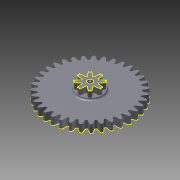
# Autodesk Inventor part: Spur Gear1
Saved by Autodesk Inventor 2014 SP1 (Build 180222100, 222)
## iProperties
Created: 2017-09-24
Part Number: Spur Gear1
Material: Steel
Document SubType Name: Modeling
Designer: Vivi
Categories: <?xml version="1.0" encoding="UTF-16"?> <MemberInstance><Categories><FamilyTemplate><FamilyTemplateParameter ValueType="xs:double" Id="1" ObjectReferenceKey="da_z" ObjectType="kUserParameterObject"/><FamilyTemplateParameter ValueType="xs:double" Id="2" ObjectReferenceKey="da_b" ObjectType="kUserParameterObject"/><FamilyTemplateParameter ValueType="xs:double" Id="3" ObjectReferenceKey="da_beta" ObjectType="kUserParameterObject"/><FamilyTemplateParameter ValueType="xs:double" Id="4" ObjectReferenceKey="da_da" ObjectType="kUserParameterObject"/><FamilyTemplateParameter ValueType="xs:double" Id="5" ObjectReferenceKey="da_aw" ObjectType="kUserParameterObject"/><FamilyTemplateParameter ValueType="xs:string" Id="6" ObjectReferenceKey="EAIAABAAAACIAQAAAAAAAIAAAAAAAAAA" ObjectType="83910656" SubObjectId="SurfaceGeometry"/></FamilyTemplate><ParamToTemplateMap><ParamToTemplate CategoryParameter="//CategoryParameter[@InternalName='046C89C9-8512-4d59-83FE-43B91F4F132A']" TemplateParameter="1"/><ParamToTemplate CategoryParameter="//CategoryParameter[@InternalName='2552DF32-E462-4b46-AEBF-C6C7768E72AC']" TemplateParameter="2"/><ParamToTemplate CategoryParameter="//CategoryParameter[@InternalName='C9EE641D-15FC-4fae-A226-E94C4372FDD7']" TemplateParameter="3"/><ParamToTemplate><ParamToTemplate CategoryParameter="//CategoryParameter[@InternalName='00B6519A-459B-49c7-AD84-2E56D39A5744']" ConstantValue="0.000000"/></ParamToTemplate><ParamToTemplate><ParamToTemplate CategoryParameter="//CategoryParameter[@InternalName='04B31F0E-C7A6-4894-AA32-9629BEFACF47']" ConstantValue="1.000000"/></ParamToTemplate><ParamToTemplate><ParamToTemplate CategoryParameter="//CategoryParameter[@InternalName='43CBEC2E-7847-49e7-A936-2F7889FCB2D9']" ConstantValue="0.250000"/></ParamToTemplate><ParamToTemplate><ParamToTemplate CategoryParameter="//CategoryParameter[@InternalName='B1EFC894-105D-4ebd-86BF-FA20ED196853']" ConstantValue="0.350000"/></ParamToTemplate><ParamToTemplate><ParamToTemplate CategoryParameter="//CategoryParameter[@InternalName='51175063-3D10-4879-93E8-6246FE8B403D']" ConstantValue="2060000000.000000"/></ParamToTemplate><ParamToTemplate><ParamToTemplate CategoryParameter="//CategoryParameter[@InternalName='A3A52E27-4454-46a9-B0BD-C932399B70AF']" ConstantValue="0.300000"/></ParamToTemplate><ParamToTemplate><ParamToTemplate CategoryParameter="//CategoryParameter[@InternalName='91B76062-C214-41d9-B1B9-14D2AB99603D']" ConstantValue="0.150000"/></ParamToTemplate><ParamToTemplate><ParamToTemplate CategoryParameter="//CategoryParameter[@InternalName='374E806E-8B8A-4dda-A9AA-1039D6500AD2']" ConstantValue="6.666667"/></ParamToTemplate><ParamToTemplate><ParamToTemplate CategoryParameter="//CategoryParameter[@InternalName='2D373A89-B862-43d6-8D0B-0CBF12AB9F6C']" ConstantValue="0.523599"/></ParamToTemplate><ParamToTemplate CategoryParameter="//CategoryParameter[@InternalName='37777632-D6A2-4fac-9D53-DB8ACD95C989']" TemplateParameter="4"/><ParamToTemplate CategoryParameter="//CategoryParameter[@InternalName='FD1017F1-B727-4f7e-9707-0F86F1FF9423']" TemplateParameter="5"/><ParamToTemplate><ParamToTemplate CategoryParameter="//CategoryParameter[@InternalName='9E1B4470-B2D3-4ff1-B813-535BB4CDF51A']" ConstantValue="3520000.000000"/></ParamToTemplate><ParamToTemplate><ParamToTemplate CategoryParameter="//CategoryParameter[@InternalName='F8452263-BFF6-458c-9FB1-07C4B99E95CD']" ConstantValue="11400000.000000"/></ParamToTemplate><ParamToTemplate><ParamToTemplate CategoryParameter="//CategoryParameter[@InternalName='3E3BB259-FD49-497f-8171-6EBC954A3479']" ConstantValue="2.000000"/></ParamToTemplate><ParamToTemplate CategoryParameter="//CategoryParameter[@InternalName='27C3BAF2-7550-4e4b-AE2C-0DB134B7D9B7']" TemplateParameter="6"/></ParamToTemplateMap><Category DisplayName="Gear" InternalName="DC85795E-93AB-48d5-8EEE-5A27447B64BD" Mnemonic="Gear"><CategoryParameter DisplayName="z" InternalName="046C89C9-8512-4d59-83FE-43B91F4F132A" Mnemonic="z"/><CategoryParameter DisplayName="b" InternalName="2552DF32-E462-4b46-AEBF-C6C7768E72AC" Mnemonic="b"/><CategoryParameter DisplayName="||b|" InternalName="C9EE641D-15FC-4fae-A226-E94C4372FDD7" Mnemonic="beta"/><CategoryParameter DisplayName="x" InternalName="00B6519A-459B-49c7-AD84-2E56D39A5744" Mnemonic="x"/><CategoryParameter DisplayName="a*" InternalName="04B31F0E-C7A6-4894-AA32-9629BEFACF47" Mnemonic="a"/><CategoryParameter DisplayName="c*" InternalName="43CBEC2E-7847-49e7-A936-2F7889FCB2D9" Mnemonic="c"/><CategoryParameter DisplayName="r|.f|*" InternalName="B1EFC894-105D-4ebd-86BF-FA20ED196853" Mnemonic="rf"/><CategoryParameter DisplayName="E" InternalName="51175063-3D10-4879-93E8-6246FE8B403D" Mnemonic="E"/><CategoryParameter DisplayName="||m|" InternalName="A3A52E27-4454-46a9-B0BD-C932399B70AF" Mnemonic="mi"/><Category DisplayName="SpurGear" InternalName="26C5A22E-A91E-4dfd-A3B3-23CCAFAE1764" Mnemonic="SpurGear"><CategoryParameter DisplayName="m" InternalName="91B76062-C214-41d9-B1B9-14D2AB99603D" Mnemonic="m"/><CategoryParameter DisplayName="P" InternalName="374E806E-8B8A-4dda-A9AA-1039D6500AD2" Mnemonic="PP"/><CategoryParameter DisplayName="||a|" InternalName="2D373A89-B862-43d6-8D0B-0CBF12AB9F6C" Mnemonic="alpha"/><CategoryParameter DisplayName="d|.a|" InternalName="37777632-D6A2-4fac-9D53-DB8ACD95C989" Mnemonic="da"/><CategoryParameter DisplayName="a|.w|" InternalName="FD1017F1-B727-4f7e-9707-0F86F1FF9423" Mnemonic="aw"/><CategoryParameter DisplayName="||s||.Flim|" InternalName="9E1B4470-B2D3-4ff1-B813-535BB4CDF51A" Mnemonic="sFlim"/><CategoryParameter DisplayName="||s||.Hlim|" InternalName="F8452263-BFF6-458c-9FB1-07C4B99E95CD" Mnemonic="sHlim"/><CategoryParameter DisplayName="type" InternalName="3E3BB259-FD49-497f-8171-6EBC954A3479" Mnemonic="type"/><CategoryParameter DisplayName="PitchDiameter" InternalName="27C3BAF2-7550-4e4b-AE2C-0DB134B7D9B7" Mnemonic="IDS_PITCHDIAM"/></Category></Category></Categories></MemberInstance>
Density: 1 g/cm^3
Appearance: Steel
CustomPartVersion: 1
Author: Vivi
Autodesk Inventor part; units mm, degrees
sketch "Sketch1" plane through (0, 0, 0) normal (0, 0, 1) x (1, 0, 0)
  circle A0 centre (0, 0) radius 27.75
  dimension "d0" = 55.5
  constraints: 1 centre point
  measures "d0" diameter of A0
extrude "Extrusion1" add sketch "Sketch1" along normal blind 5
ref_plane "Work Plane2" through (0, 0, 2.5) normal (0, 0, 1) x (1, 0, 0)
sketch "Sketch2" plane through (0, 0, 0) normal (0, 0, -1) x (-1, 0, 0)
  circle A0 centre (0, 0) radius 27.75 projected
  circle A1 centre (0, 0) radius 26.25
  dimension "d3" = 52.5
  constraints: 1 centre point, 1 coincident
  measures "d3" diameter of A1
surface extrude "Pitch Diameter" sketch "Sketch2" against normal through all shown no curves A1
ref_plane "Work Plane8" through (0, 0, 0) normal (0.9959743, 0.0896393, 0) x (0, 0, 1)
ref_plane "Work Plane9" through (0, 0, 0) normal (1, 0, 0) x (0, 1, 0)
spur gear teeth "Spur Gear" teeth 35 pitch diameter 52.5 tip diameter 55.5 root diameter 48.75 face width 10 start plane through (0, 0, 0) normal (0, 0, -1) x (-1, 0, 0)
sketch "Sketch3" plane through (0, 0, 5) normal (0, 0, 1) x (1, 0, 0)
  circle A0 centre (0, 0) radius 1.1
  arc A1 (3.6379, 1.9445) -> (5.7976, 4.7579) centre (-0.6751, 7.4909) ccw
  arc A2 (5.7976, 4.7579) -> (4.7579, 5.7976) centre (0, 0) ccw
  arc A3 (4.7579, 5.7976) -> (1.9445, 3.6379) centre (7.4909, -0.6751) ccw
  arc A4 (1.9445, 3.6379) -> (1.1974, 3.9474) centre (0, 0) ccw
  arc A5 (1.1974, 3.9474) -> (0.7351, 7.4639) centre (-5.7742, 4.8195) ccw
  arc A6 (0.7351, 7.4639) -> (-0.7351, 7.4639) centre (0, 0) ccw
  arc A7 (-0.7351, 7.4639) -> (-1.1974, 3.9474) centre (5.7742, 4.8195) ccw
  arc A8 (-1.1974, 3.9474) -> (-1.9445, 3.6379) centre (0, 0) ccw
  arc A9 (-1.9445, 3.6379) -> (-4.7579, 5.7976) centre (-7.4909, -0.6751) ccw
  arc A10 (-4.7579, 5.7976) -> (-5.7976, 4.7579) centre (0, 0) ccw
  arc A11 (-5.7976, 4.7579) -> (-3.6379, 1.9445) centre (0.6751, 7.4909) ccw
  arc A12 (-3.6379, 1.9445) -> (-3.9474, 1.1974) centre (0, 0) ccw
  arc A13 (-3.9474, 1.1974) -> (-7.4639, 0.7351) centre (-4.8195, -5.7742) ccw
  arc A14 (-7.4639, 0.7351) -> (-7.4639, -0.7351) centre (0, 0) ccw
  arc A15 (-7.4639, -0.7351) -> (-3.9474, -1.1974) centre (-4.8195, 5.7742) ccw
  arc A16 (-3.9474, -1.1974) -> (-3.6379, -1.9445) centre (0, 0) ccw
  arc A17 (-3.6379, -1.9445) -> (-5.7976, -4.7579) centre (0.6751, -7.4909) ccw
  arc A18 (-5.7976, -4.7579) -> (-4.7579, -5.7976) centre (0, 0) ccw
  arc A19 (-4.7579, -5.7976) -> (-1.9445, -3.6379) centre (-7.4909, 0.6751) ccw
  arc A20 (-1.9445, -3.6379) -> (-1.1974, -3.9474) centre (0, 0) ccw
  arc A21 (-1.1974, -3.9474) -> (-0.7351, -7.4639) centre (5.7742, -4.8195) ccw
  arc A22 (-0.7351, -7.4639) -> (0.7351, -7.4639) centre (0, 0) ccw
  arc A23 (0.7351, -7.4639) -> (1.1974, -3.9474) centre (-5.7742, -4.8195) ccw
  arc A24 (1.1974, -3.9474) -> (1.9445, -3.6379) centre (0, 0) ccw
  arc A25 (1.9445, -3.6379) -> (4.7579, -5.7976) centre (7.4909, 0.6751) ccw
  arc A26 (4.7579, -5.7976) -> (5.7976, -4.7579) centre (0, 0) ccw
  arc A27 (5.7976, -4.7579) -> (3.6379, -1.9445) centre (-0.6751, -7.4909) ccw
  arc A28 (3.6379, -1.9445) -> (3.9474, -1.1974) centre (0, 0) ccw
  arc A29 (3.9474, -1.1974) -> (7.4639, -0.7351) centre (4.8195, 5.7742) ccw
  arc A30 (7.4639, -0.7351) -> (7.4639, 0.7351) centre (0, 0) ccw
  arc A31 (7.4639, 0.7351) -> (3.9474, 1.1974) centre (4.8195, -5.7742) ccw
  arc A32 (3.9474, 1.1974) -> (3.6379, 1.9445) centre (0, 0) ccw
  circle A33 centre (0, 0) radius 1.75
  dimension "d49" = 3.5
  constraints: 64 point on circle, 34 centre point, 1 coincident
  measures "d49" diameter of A33
extrude "Extrusion2" add sketch "Sketch3" along normal blind 5 contours A32 A31 A30 A29 A28 A27 A26 A25 A24 A23 A22 A21 A20 A19 A18 A17 A16 A15 A14 A13 A12 A11 A10 A9 A8 A7 A6 A5 A4 A3 A2 A1
sketch "Sketch4" plane through (0, 0, 5) normal (0, 0, 1) x (1, 0, 0)
  circle A0 centre (0, 0) radius 1.75 projected
extrude "Extrusion3" cut sketch "Sketch4" against normal blind 10
sketch "Sketch6" plane through (0, 0, 5) normal (0, 0, 1) x (1, 0, 0)
  arc A0 (0.7351, 7.4639) -> (-0.7351, 7.4639) centre (0, 0) ccw projected
  arc A1 (1.1974, 3.9474) -> (0.7351, 7.4639) centre (-5.7742, 4.8195) ccw projected
  arc A2 (1.9445, 3.6379) -> (1.1974, 3.9474) centre (0, 0) ccw projected
  arc A3 (4.7579, 5.7976) -> (1.9445, 3.6379) centre (7.4909, -0.6751) ccw projected
  arc A4 (5.7976, 4.7579) -> (4.7579, 5.7976) centre (0, 0) ccw projected
  arc A5 (3.6379, 1.9445) -> (5.7976, 4.7579) centre (-0.6751, 7.4909) ccw projected
  arc A6 (3.9474, 1.1974) -> (3.6379, 1.9445) centre (0, 0) ccw projected
  arc A7 (7.4639, 0.7351) -> (3.9474, 1.1974) centre (4.8195, -5.7742) ccw projected
  arc A8 (7.4639, -0.7351) -> (7.4639, 0.7351) centre (0, 0) ccw projected
  arc A9 (3.9474, -1.1974) -> (7.4639, -0.7351) centre (4.8195, 5.7742) ccw projected
  arc A10 (3.6379, -1.9445) -> (3.9474, -1.1974) centre (0, 0) ccw projected
  arc A11 (5.7976, -4.7579) -> (3.6379, -1.9445) centre (-0.6751, -7.4909) ccw projected
  arc A12 (4.7579, -5.7976) -> (5.7976, -4.7579) centre (0, 0) ccw projected
  arc A13 (1.9445, -3.6379) -> (4.7579, -5.7976) centre (7.4909, 0.6751) ccw projected
  arc A14 (1.1974, -3.9474) -> (1.9445, -3.6379) centre (0, 0) ccw projected
  arc A15 (0.7351, -7.4639) -> (1.1974, -3.9474) centre (-5.7742, -4.8195) ccw projected
  arc A16 (-0.7351, -7.4639) -> (0.7351, -7.4639) centre (0, 0) ccw projected
  arc A17 (-1.1974, -3.9474) -> (-0.7351, -7.4639) centre (5.7742, -4.8195) ccw projected
  arc A18 (-1.9445, -3.6379) -> (-1.1974, -3.9474) centre (0, 0) ccw projected
  arc A19 (-4.7579, -5.7976) -> (-1.9445, -3.6379) centre (-7.4909, 0.6751) ccw projected
  arc A20 (-5.7976, -4.7579) -> (-4.7579, -5.7976) centre (0, 0) ccw projected
  arc A21 (-3.6379, -1.9445) -> (-5.7976, -4.7579) centre (0.6751, -7.4909) ccw projected
  arc A22 (-3.9474, -1.1974) -> (-3.6379, -1.9445) centre (0, 0) ccw projected
  arc A23 (-7.4639, -0.7351) -> (-3.9474, -1.1974) centre (-4.8195, 5.7742) ccw projected
  arc A24 (-7.4639, 0.7351) -> (-7.4639, -0.7351) centre (0, 0) ccw projected
  arc A25 (-3.9474, 1.1974) -> (-7.4639, 0.7351) centre (-4.8195, -5.7742) ccw projected
  arc A26 (-3.6379, 1.9445) -> (-3.9474, 1.1974) centre (0, 0) ccw projected
  arc A27 (-5.7976, 4.7579) -> (-3.6379, 1.9445) centre (0.6751, 7.4909) ccw projected
  arc A28 (-4.7579, 5.7976) -> (-5.7976, 4.7579) centre (0, 0) ccw projected
  arc A29 (-1.9445, 3.6379) -> (-4.7579, 5.7976) centre (-7.4909, -0.6751) ccw projected
  arc A30 (-1.1974, 3.9474) -> (-1.9445, 3.6379) centre (0, 0) ccw projected
  arc A31 (-0.7351, 7.4639) -> (-1.1974, 3.9474) centre (5.7742, 4.8195) ccw projected
  circle A32 centre (0, 0) radius 8
  dimension "d54" = 16
  constraints: 1 centre point, 1 coincident
  measures "d54" diameter of A32
extrude "Extrusion4" add sketch "Sketch6" along normal blind 1
fillet "Fillet1" radius 1 1 edges at (-8, 0, 5)
sketch "Sketch7" plane through (0, 0, 0) normal (0, 0, -1) x (-1, 0, 0)
  circle A0 centre (0, 0) radius 1.75 projected
  arc A1 (5.9558, 23.6362) -> (5.5664, 27.186) centre (-9.9956, 23.6825) ccw projected
  arc A2 (5.5664, 27.186) -> (4.3411, 27.4084) centre (0, 0) ccw projected
  arc A3 (4.3411, 27.4084) -> (2.7291, 24.2217) centre (17.6796, 18.6602) ccw projected
  arc A4 (2.7291, 24.2217) -> (1.6397, 24.3198) centre (0, 0) ccw projected
  arc A5 (1.6397, 24.3198) -> (0.6227, 27.743) centre (-14.0636, 21.5171) ccw projected
  arc A6 (0.6227, 27.743) -> (-0.6227, 27.743) centre (0, 0) ccw projected
  arc A7 (-0.6227, 27.743) -> (-1.6397, 24.3198) centre (14.0636, 21.5171) ccw projected
  arc A8 (-1.6397, 24.3198) -> (-2.7291, 24.2217) centre (0, 0) ccw projected
  arc A9 (-2.7291, 24.2217) -> (-4.3411, 27.4084) centre (-17.6796, 18.6602) ccw projected
  arc A10 (-4.3411, 27.4084) -> (-5.5664, 27.186) centre (0, 0) ccw projected
  arc A11 (-5.5664, 27.186) -> (-5.9558, 23.6362) centre (9.9956, 23.6825) ccw projected
  arc A12 (-5.9558, 23.6362) -> (-7.0102, 23.3452) centre (0, 0) ccw projected
  arc A13 (-7.0102, 23.3452) -> (-9.1652, 26.1928) centre (-20.7274, 15.2035) ccw projected
  arc A14 (-9.1652, 26.1928) -> (-10.3311, 25.7552) centre (0, 0) ccw projected
  arc A15 (-10.3311, 25.7552) -> (-10.0805, 22.1929) centre (5.6063, 25.0867) ccw projected
  arc A16 (-10.0805, 22.1929) -> (-11.066, 21.7183) centre (0, 0) ccw projected
  arc A17 (-11.066, 21.7183) -> (-13.6949, 24.1353) centre (-23.109, 11.2581) ccw projected
  arc A18 (-13.6949, 24.1353) -> (-14.7639, 23.4966) centre (0, 0) ccw projected
  arc A19 (-14.7639, 23.4966) -> (-13.8812, 20.0363) centre (1.0368, 25.6845) ccw projected
  arc A20 (-13.8812, 20.0363) -> (-14.7661, 19.3933) centre (0, 0) ccw projected
  arc A21 (-14.7661, 19.3933) -> (-17.7843, 21.3021) centre (-24.7478, 6.9509) ccw projected
  arc A22 (-17.7843, 21.3021) -> (-18.7221, 20.4828) centre (0, 0) ccw projected
  arc A23 (-18.7221, 20.4828) -> (-17.2357, 17.2357) centre (-3.566, 25.4569) ccw projected
  arc A24 (-17.2357, 17.2357) -> (-17.9917, 16.4451) centre (0, 0) ccw projected
  arc A25 (-17.9917, 16.4451) -> (-21.3021, 17.7843) centre (-25.5913, 2.4203) ccw projected
  arc A26 (-21.3021, 17.7843) -> (-22.0786, 16.8107) centre (0, 0) ccw projected
  arc A27 (-22.0786, 16.8107) -> (-20.0363, 13.8812) centre (-8.0542, 24.4111) ccw projected
  arc A28 (-20.0363, 13.8812) -> (-20.6389, 12.9683) centre (0, 0) ccw projected
  arc A29 (-20.6389, 12.9683) -> (-24.1353, 13.6949) centre (-25.6122, -2.1881) ccw projected
  arc A30 (-24.1353, 13.6949) -> (-24.7254, 12.5982) centre (0, 0) ccw projected
  arc A31 (-24.7254, 12.5982) -> (-22.1929, 10.0805) centre (-12.2836, 22.5806) ccw projected
  arc A32 (-22.1929, 10.0805) -> (-22.6228, 9.0747) centre (0, 0) ccw projected
  arc A33 (-22.6228, 9.0747) -> (-26.1928, 9.1652) centre (-24.8099, -6.7261) ccw projected
  arc A34 (-26.1928, 9.1652) -> (-26.5776, 7.9809) centre (0, 0) ccw projected
  arc A35 (-26.5776, 7.9809) -> (-23.6362, 5.9558) centre (-16.1181, 20.0244) ccw projected
  arc A36 (-23.6362, 5.9558) -> (-23.8796, 4.8894) centre (0, 0) ccw projected
  arc A37 (-23.8796, 4.8894) -> (-27.4084, 4.3411) centre (-23.2102, -11.048) ccw projected
  arc A38 (-27.4084, 4.3411) -> (-27.5755, 3.107) centre (0, 0) ccw projected
  arc A39 (-27.5755, 3.107) -> (-24.3198, 1.6397) centre (-19.4346, 16.8246) ccw projected
  arc A40 (-24.3198, 1.6397) -> (-24.3689, 0.5469) centre (0, 0) ccw projected
  arc A41 (-24.3689, 0.5469) -> (-27.743, -0.6227) centre (-20.8645, -15.0148) ccw projected
  arc A42 (-27.743, -0.6227) -> (-27.6871, -1.8667) centre (0, 0) ccw projected
  arc A43 (-27.6871, -1.8667) -> (-24.2217, -2.7291) centre (-22.1264, 13.0841) ccw projected
  arc A44 (-24.2217, -2.7291) -> (-24.0749, -3.8131) centre (0, 0) ccw projected
  arc A45 (-24.0749, -3.8131) -> (-27.186, -5.5664) centre (-17.8482, -18.499) ccw projected
  arc A46 (-27.186, -5.5664) -> (-26.9089, -6.7804) centre (0, 0) ccw projected
  arc A47 (-26.9089, -6.7804) -> (-23.3452, -7.0102) centre (-24.1071, 8.923) ccw projected
  arc A48 (-23.3452, -7.0102) -> (-23.0072, -8.0506) centre (0, 0) ccw projected
  arc A49 (-23.0072, -8.0506) -> (-25.7552, -10.3311) centre (-14.2582, -21.3886) ccw projected
  arc A50 (-25.7552, -10.3311) -> (-25.2658, -11.4762) centre (0, 0) ccw projected
  arc A51 (-25.2658, -11.4762) -> (-21.7183, -11.066) centre (-25.3129, 4.4751) ccw projected
  arc A52 (-21.7183, -11.066) -> (-21.1999, -12.0293) centre (0, 0) ccw projected
  arc A53 (-21.1999, -12.0293) -> (-23.4966, -14.7639) centre (-10.21, -23.5908) ccw projected
  arc A54 (-23.4966, -14.7639) -> (-22.8106, -15.8032) centre (0, 0) ccw projected
  arc A55 (-22.8106, -15.8032) -> (-19.3933, -14.7661) centre (-25.7052, -0.1166) ccw projected
  arc A56 (-19.3933, -14.7661) -> (-18.7113, -15.6213) centre (0, 0) ccw projected
  arc A57 (-18.7113, -15.6213) -> (-20.4828, -18.7221) centre (-5.8336, -25.0348) ccw projected
  arc A58 (-20.4828, -18.7221) -> (-19.6222, -19.6222) centre (0, 0) ccw projected
  arc A59 (-19.6222, -19.6222) -> (-16.4451, -17.9917) centre (-25.2713, -4.7046) ccw projected
  arc A60 (-16.4451, -17.9917) -> (-15.6213, -18.7113) centre (0, 0) ccw projected
  arc A61 (-15.6213, -18.7113) -> (-16.8107, -22.0786) centre (-1.2697, -25.6741) ccw projected
  arc A62 (-16.8107, -22.0786) -> (-15.8032, -22.8106) centre (0, 0) ccw projected
  arc A63 (-15.8032, -22.8106) -> (-12.9683, -20.6389) centre (-24.0251, -9.1413) ccw projected
  arc A64 (-12.9683, -20.6389) -> (-12.0293, -21.1999) centre (0, 0) ccw projected
  arc A65 (-12.0293, -21.1999) -> (-12.5982, -24.7254) centre (3.335, -25.4882) ccw projected
  arc A66 (-12.5982, -24.7254) -> (-11.4762, -25.2658) centre (0, 0) ccw projected
  arc A67 (-11.4762, -25.2658) -> (-9.0747, -22.6228) centre (-22.0068, -13.2843) ccw projected
  arc A68 (-9.0747, -22.6228) -> (-8.0506, -23.0072) centre (0, 0) ccw projected
  arc A69 (-8.0506, -23.0072) -> (-7.9809, -26.5776) centre (7.8325, -24.4831) ccw projected
  arc A70 (-7.9809, -26.5776) -> (-6.7804, -26.9089) centre (0, 0) ccw projected
  arc A71 (-6.7804, -26.9089) -> (-4.8894, -23.8796) centre (-19.2811, -17.0002) ccw projected
  arc A72 (-4.8894, -23.8796) -> (-3.8131, -24.0749) centre (0, 0) ccw projected
  arc A73 (-3.8131, -24.0749) -> (-3.107, -27.5755) centre (12.0782, -22.6911) ccw projected
  arc A74 (-3.107, -27.5755) -> (-1.8667, -27.6871) centre (0, 0) ccw projected
  arc A75 (-1.8667, -27.6871) -> (-0.5469, -24.3689) centre (-15.9358, -20.1698) ccw projected
  arc A76 (-0.5469, -24.3689) -> (0.5469, -24.3689) centre (0, 0) ccw projected
  arc A77 (0.5469, -24.3689) -> (1.8667, -27.6871) centre (15.9358, -20.1698) ccw projected
  arc A78 (1.8667, -27.6871) -> (3.107, -27.5755) centre (0, 0) ccw projected
  arc A79 (3.107, -27.5755) -> (3.8131, -24.0749) centre (-12.0782, -22.6911) ccw projected
  arc A80 (3.8131, -24.0749) -> (4.8894, -23.8796) centre (0, 0) ccw projected
  arc A81 (4.8894, -23.8796) -> (6.7804, -26.9089) centre (19.2811, -17.0002) ccw projected
  arc A82 (6.7804, -26.9089) -> (7.9809, -26.5776) centre (0, 0) ccw projected
  arc A83 (7.9809, -26.5776) -> (8.0506, -23.0072) centre (-7.8325, -24.4831) ccw projected
  arc A84 (8.0506, -23.0072) -> (9.0747, -22.6228) centre (0, 0) ccw projected
  arc A85 (9.0747, -22.6228) -> (11.4762, -25.2658) centre (22.0068, -13.2843) ccw projected
  arc A86 (11.4762, -25.2658) -> (12.5982, -24.7254) centre (0, 0) ccw projected
  arc A87 (12.5982, -24.7254) -> (12.0293, -21.1999) centre (-3.335, -25.4882) ccw projected
  arc A88 (12.0293, -21.1999) -> (12.9683, -20.6389) centre (0, 0) ccw projected
  arc A89 (12.9683, -20.6389) -> (15.8032, -22.8106) centre (24.0251, -9.1413) ccw projected
  arc A90 (15.8032, -22.8106) -> (16.8107, -22.0786) centre (0, 0) ccw projected
  arc A91 (16.8107, -22.0786) -> (15.6213, -18.7113) centre (1.2697, -25.6741) ccw projected
  arc A92 (15.6213, -18.7113) -> (16.4451, -17.9917) centre (0, 0) ccw projected
  arc A93 (16.4451, -17.9917) -> (19.6222, -19.6222) centre (25.2713, -4.7046) ccw projected
  arc A94 (19.6222, -19.6222) -> (20.4828, -18.7221) centre (0, 0) ccw projected
  arc A95 (20.4828, -18.7221) -> (18.7113, -15.6213) centre (5.8336, -25.0348) ccw projected
  arc A96 (18.7113, -15.6213) -> (19.3933, -14.7661) centre (0, 0) ccw projected
  arc A97 (19.3933, -14.7661) -> (22.8106, -15.8032) centre (25.7052, -0.1166) ccw projected
  arc A98 (22.8106, -15.8032) -> (23.4966, -14.7639) centre (0, 0) ccw projected
  arc A99 (23.4966, -14.7639) -> (21.1999, -12.0293) centre (10.21, -23.5908) ccw projected
  arc A100 (21.1999, -12.0293) -> (21.7183, -11.066) centre (0, 0) ccw projected
  arc A101 (21.7183, -11.066) -> (25.2658, -11.4762) centre (25.3129, 4.4751) ccw projected
  arc A102 (25.2658, -11.4762) -> (25.7552, -10.3311) centre (0, 0) ccw projected
  arc A103 (25.7552, -10.3311) -> (23.0072, -8.0506) centre (14.2582, -21.3886) ccw projected
  arc A104 (23.0072, -8.0506) -> (23.3452, -7.0102) centre (0, 0) ccw projected
  arc A105 (23.3452, -7.0102) -> (26.9089, -6.7804) centre (24.1071, 8.923) ccw projected
  arc A106 (26.9089, -6.7804) -> (27.186, -5.5664) centre (0, 0) ccw projected
  arc A107 (27.186, -5.5664) -> (24.0749, -3.8131) centre (17.8482, -18.499) ccw projected
  arc A108 (24.0749, -3.8131) -> (24.2217, -2.7291) centre (0, 0) ccw projected
  arc A109 (24.2217, -2.7291) -> (27.6871, -1.8667) centre (22.1264, 13.0841) ccw projected
  arc A110 (27.6871, -1.8667) -> (27.743, -0.6227) centre (0, 0) ccw projected
  arc A111 (27.743, -0.6227) -> (24.3689, 0.5469) centre (20.8645, -15.0148) ccw projected
  arc A112 (24.3689, 0.5469) -> (24.3198, 1.6397) centre (0, 0) ccw projected
  arc A113 (24.3198, 1.6397) -> (27.5755, 3.107) centre (19.4346, 16.8246) ccw projected
  arc A114 (27.5755, 3.107) -> (27.4084, 4.3411) centre (0, 0) ccw projected
  arc A115 (27.4084, 4.3411) -> (23.8796, 4.8894) centre (23.2102, -11.048) ccw projected
  arc A116 (23.8796, 4.8894) -> (23.6362, 5.9558) centre (0, 0) ccw projected
  arc A117 (23.6362, 5.9558) -> (26.5776, 7.9809) centre (16.1181, 20.0244) ccw projected
  arc A118 (26.5776, 7.9809) -> (26.1928, 9.1652) centre (0, 0) ccw projected
  arc A119 (26.1928, 9.1652) -> (22.6228, 9.0747) centre (24.8099, -6.7261) ccw projected
  arc A120 (22.6228, 9.0747) -> (22.1929, 10.0805) centre (0, 0) ccw projected
  arc A121 (22.1929, 10.0805) -> (24.7254, 12.5982) centre (12.2836, 22.5806) ccw projected
  arc A122 (24.7254, 12.5982) -> (24.1353, 13.6949) centre (0, 0) ccw projected
  arc A123 (24.1353, 13.6949) -> (20.6389, 12.9683) centre (25.6122, -2.1881) ccw projected
  arc A124 (20.6389, 12.9683) -> (20.0363, 13.8812) centre (0, 0) ccw projected
  arc A125 (20.0363, 13.8812) -> (22.0786, 16.8107) centre (8.0542, 24.4111) ccw projected
  arc A126 (22.0786, 16.8107) -> (21.3021, 17.7843) centre (0, 0) ccw projected
  arc A127 (21.3021, 17.7843) -> (17.9917, 16.4451) centre (25.5913, 2.4203) ccw projected
  arc A128 (17.9917, 16.4451) -> (17.2357, 17.2357) centre (0, 0) ccw projected
  arc A129 (17.2357, 17.2357) -> (18.7221, 20.4828) centre (3.566, 25.4569) ccw projected
  arc A130 (18.7221, 20.4828) -> (17.7843, 21.3021) centre (0, 0) ccw projected
  arc A131 (17.7843, 21.3021) -> (14.7661, 19.3933) centre (24.7478, 6.9509) ccw projected
  arc A132 (14.7661, 19.3933) -> (13.8812, 20.0363) centre (0, 0) ccw projected
  arc A133 (13.8812, 20.0363) -> (14.7639, 23.4966) centre (-1.0368, 25.6845) ccw projected
  arc A134 (14.7639, 23.4966) -> (13.6949, 24.1353) centre (0, 0) ccw projected
  arc A135 (13.6949, 24.1353) -> (11.066, 21.7183) centre (23.109, 11.2581) ccw projected
  arc A136 (11.066, 21.7183) -> (10.0805, 22.1929) centre (0, 0) ccw projected
  arc A137 (10.0805, 22.1929) -> (10.3311, 25.7552) centre (-5.6063, 25.0867) ccw projected
  arc A138 (10.3311, 25.7552) -> (9.1652, 26.1928) centre (0, 0) ccw projected
  arc A139 (9.1652, 26.1928) -> (7.0102, 23.3452) centre (20.7274, 15.2035) ccw projected
  arc A140 (7.0102, 23.3452) -> (5.9558, 23.6362) centre (0, 0) ccw projected
sketch "Sketch8" plane through (0, 0, 10) normal (0, 0, 1) x (1, 0, 0)
  circle A0 centre (0, 0) radius 1.75 projected
  arc A1 (-0.7351, 7.4639) -> (-1.1974, 3.9474) centre (5.7742, 4.8195) ccw projected
  arc A2 (-1.1974, 3.9474) -> (-1.9445, 3.6379) centre (0, 0) ccw projected
  arc A3 (-1.9445, 3.6379) -> (-4.7579, 5.7976) centre (-7.4909, -0.6751) ccw projected
  arc A4 (-4.7579, 5.7976) -> (-5.7976, 4.7579) centre (0, 0) ccw projected
  arc A5 (-5.7976, 4.7579) -> (-3.6379, 1.9445) centre (0.6751, 7.4909) ccw projected
  arc A6 (-3.6379, 1.9445) -> (-3.9474, 1.1974) centre (0, 0) ccw projected
  arc A7 (-3.9474, 1.1974) -> (-7.4639, 0.7351) centre (-4.8195, -5.7742) ccw projected
  arc A8 (-7.4639, 0.7351) -> (-7.4639, -0.7351) centre (0, 0) ccw projected
  arc A9 (-7.4639, -0.7351) -> (-3.9474, -1.1974) centre (-4.8195, 5.7742) ccw projected
  arc A10 (-3.9474, -1.1974) -> (-3.6379, -1.9445) centre (0, 0) ccw projected
  arc A11 (-3.6379, -1.9445) -> (-5.7976, -4.7579) centre (0.6751, -7.4909) ccw projected
  arc A12 (-5.7976, -4.7579) -> (-4.7579, -5.7976) centre (0, 0) ccw projected
  arc A13 (-4.7579, -5.7976) -> (-1.9445, -3.6379) centre (-7.4909, 0.6751) ccw projected
  arc A14 (-1.9445, -3.6379) -> (-1.1974, -3.9474) centre (0, 0) ccw projected
  arc A15 (-1.1974, -3.9474) -> (-0.7351, -7.4639) centre (5.7742, -4.8195) ccw projected
  arc A16 (-0.7351, -7.4639) -> (0.7351, -7.4639) centre (0, 0) ccw projected
  arc A17 (0.7351, -7.4639) -> (1.1974, -3.9474) centre (-5.7742, -4.8195) ccw projected
  arc A18 (1.1974, -3.9474) -> (1.9445, -3.6379) centre (0, 0) ccw projected
  arc A19 (1.9445, -3.6379) -> (4.7579, -5.7976) centre (7.4909, 0.6751) ccw projected
  arc A20 (4.7579, -5.7976) -> (5.7976, -4.7579) centre (0, 0) ccw projected
  arc A21 (5.7976, -4.7579) -> (3.6379, -1.9445) centre (-0.6751, -7.4909) ccw projected
  arc A22 (3.6379, -1.9445) -> (3.9474, -1.1974) centre (0, 0) ccw projected
  arc A23 (3.9474, -1.1974) -> (7.4639, -0.7351) centre (4.8195, 5.7742) ccw projected
  arc A24 (7.4639, -0.7351) -> (7.4639, 0.7351) centre (0, 0) ccw projected
  arc A25 (7.4639, 0.7351) -> (3.9474, 1.1974) centre (4.8195, -5.7742) ccw projected
  arc A26 (3.9474, 1.1974) -> (3.6379, 1.9445) centre (0, 0) ccw projected
  arc A27 (3.6379, 1.9445) -> (5.7976, 4.7579) centre (-0.6751, 7.4909) ccw projected
  arc A28 (5.7976, 4.7579) -> (4.7579, 5.7976) centre (0, 0) ccw projected
  arc A29 (4.7579, 5.7976) -> (1.9445, 3.6379) centre (7.4909, -0.6751) ccw projected
  arc A30 (1.9445, 3.6379) -> (1.1974, 3.9474) centre (0, 0) ccw projected
  arc A31 (1.1974, 3.9474) -> (0.7351, 7.4639) centre (-5.7742, 4.8195) ccw projected
  arc A32 (0.7351, 7.4639) -> (-0.7351, 7.4639) centre (0, 0) ccw projected
equation "\"d0\" = da_da"
equation "\"d3\" = da_dw"
equation "\"d16\" = da_aw"
equation "\"d43\" = da_aw"
equation "\"d46\" = da_aw"
equation "\"da_da\" = 55.5"
equation "\"da_dw\" = 52.5"
equation "\"da_aw\" = 222.75"
body "Solid1"
body "Srf1"
